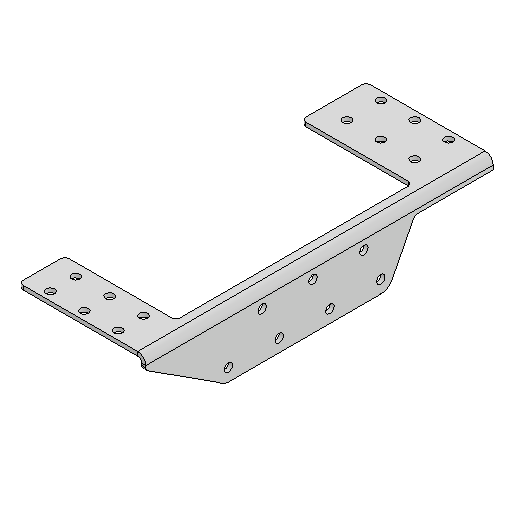
# Autodesk Inventor part: MainDriveMotorToPlateConnector
Saved by Autodesk Inventor 2025 (Build 290162000, 162)
## iProperties
Created: 2024-04-02
Part Number: MainDriveMotorToPlateConnector
Material: Generic
Document SubType Name: Sheet Metal
Designer: seene
Density: 1 g/cm^3
Sheet Metal Rule: Default
Appearance: Default
Mass: 54.1937 g
Surface Area: 394.583 cm^2
Volume: 54.1937 cm^3
Author: seene
Autodesk Inventor part; units mm, degrees
note: some values were not read from the file. Chosen so that the rebuilt part matches the saved one: flange form of "Plate2".
ref_plane "YZ Plane" through (0, 0, 0) normal (1, 0, 0) x (0, 1, 0)
ref_plane "XZ Plane" through (0, 0, 0) normal (0, 1, 0) x (-1, 0, 0)
ref_plane "XY Plane" through (0, 0, 0) normal (0, 0, 1) x (1, 0, 0)
sketch "Sketch1" plane through (0, 0, 0) normal (0, 1, 0) x (-1, 0, 0)
  line L0 (0, 0) -> (95.25, 0)
  line L1 (95.25, 0) -> (95.25, -260.35)
  line L2 (95.25, -260.35) -> (0, -260.35)
  line L3 (0, -260.35) -> (0, 0)
  circle A0 centre (77.8624, -6.35) radius 3.175
  circle A1 centre (77.8624, -25.4) radius 3.175
  circle A2 centre (52.4624, -6.35) radius 3.175
  circle A3 centre (52.4624, -25.4) radius 3.175
  circle A4 centre (27.0624, -6.35) radius 3.175
  circle A5 centre (27.0624, -25.4) radius 3.175
  circle A6 centre (77.8624, -228.6) radius 3.175
  circle A7 centre (77.8624, -254) radius 3.175
  circle A8 centre (52.4624, -228.6) radius 3.175
  circle A9 centre (52.4624, -254) radius 3.175
  circle A10 centre (27.0624, -228.6) radius 3.175
  circle A11 centre (27.0624, -254) radius 3.175
  line L4 (101.24, -208.719) -> (15.24, -208.719) construction
  line L5 (15.24, -208.719) -> (15.24, -37.719) construction
  line L6 (15.24, -37.719) -> (101.24, -37.719) construction
  line L7 (101.24, -37.719) -> (101.24, -208.719) construction
  line L8 (95.25, -211.894) -> (12.065, -211.894)
  line L9 (12.065, -211.894) -> (12.065, -34.544)
  line L10 (12.065, -34.544) -> (95.25, -34.544)
  dimension "d0" = 95.25
  dimension "d2" = 6.35
  dimension "d3" = 6.35
  dimension "d4" = 17.3876
  dimension "d7" = 19.05
  dimension "d10" = 25.4
  dimension "d15" = 25.4
  dimension "d18" = 25.4
  dimension "d21" = 222.25
  dimension "d22" = 6.35
  dimension "d54" = 86
  dimension "d55" = 177.35
  dimension "d56" = 171
  dimension "d57" = 3.175
  dimension "d58" = 34.544
  dimension "d59" = 3.175
  dimension "d60" = 12.065
  measures "d0" distance of L1.end L2.end
  measures "d2" diameter of A0
  measures "d3" distance from line of A0.centre L0
  measures "d4" distance from line of L1 A0.centre
  measures "d7" distance of A0.centre A1.centre
  measures "d10" distance of A0.centre A2.centre
  measures "d15" distance of A6.centre A7.centre
  measures "d18" distance of A6.centre A8.centre
  measures "d21" distance of A6.centre A0.centre
  measures "d22" distance from line of L2 A7.centre
  measures "d54" distance between parallel lines of L5 L7
  measures "d55" distance of L8.end L9.end
  measures "d56" distance of L4.end L5.end
  measures "d57" distance between parallel lines of L4 L8
  measures "d58" distance between parallel lines of L0 L10
  measures "d59" distance between parallel lines of L9 L5
  measures "d60" distance between parallel lines of L3 L9
extrude "Plate1" add sketch "Sketch1" along normal blind 3.048 contours L0 L1 L10 L9 L8 L2 L3
sketch "Sketch2" plane through (-3.048, 3.048, 0) normal (1, 0, 0) x (0, 1, 0)
  line L0 (0, -260.35) -> (0, 0)
  line L1 (0, 0) -> (-50.8, 0)
  line L2 (-50.8, 0) -> (-50.8, -260.35)
  line L3 (-50.8, -260.35) -> (0, -260.35)
  constraints: 6 end point, 1 horizontal, 1 perpendicular, 1 vertical
edge flange "Flange1" height 50.8 angle 90 thickness 3.048 bend radius 3.048 thickness toward (1, 0, 0) relief tear relief width 3.048 relief depth 1.524 edges at (0, 0, -130.175) wall of the first edge with corners at (-3.048, 3.048, -260.35) (-3.048, 3.048, 0) (-3.048, -47.752, 0) (-3.048, -47.752, -260.35)
bend "Bend1"
corner "Corner1"
sketch "Sketch3" plane through (0, -47.752, 0) normal (1, 0, 0) x (0, 0, -1)
  circle A0 centre (87.2198, 37.9611) radius 3.175
  circle A1 centre (61.8198, 12.5611) radius 3.175
  line L0 (0, 0) -> (0, 44.704) projected
  line L1 (260.35, 0) -> (0, 0) projected
  circle A2 centre (99.9198, 12.5611) radius 3.175
  circle A3 centre (138.0198, 12.5611) radius 3.175
  circle A4 centre (176.1198, 12.5611) radius 3.175
  circle A5 centre (125.3198, 37.9611) radius 3.175
  circle A6 centre (163.4198, 37.9611) radius 3.175
  circle A7 centre (61.8198, 12.5611) radius 9.525
  circle A8 centre (176.1198, 12.5611) radius 9.525
  line L2 (61.8198, 3.0361) -> (176.1198, 3.0361)
  line L3 (0, 44.704) -> (260.35, 44.704) projected
  line L4 (260.35, 44.704) -> (260.35, 0) projected
  line L5 (54.3999, 6.5886) -> (0, 41.529)
  line L6 (184.6703, 8.3641) -> (201.5198, 41.529)
  line L7 (201.5198, 41.529) -> (260.35, 41.529)
  point P0 (0, 47.752)
  point P1 (178.7879, 44.704)
  dimension "d34" = 6.35
  dimension "d35" = 25.4
  dimension "d36" = 25.4
  dimension "d37" = 61.8198
  dimension "d40" = 38.1
  dimension "d47" = 38.1
  dimension "d61" = 6.35
  dimension "d62" = 6.35
  dimension "d64" = 3.175
  dimension "d65" = 3.175
  dimension "d66" = 25.4
  constraints: 9 centre point, 8 end point, 4 point on circle, 3 horizontal, 3 point on line, 1 equal radius, 1 parallel, 10 other
  measures "d34" diameter of A0
  measures "d35" horizontal distance of A0.centre A1.centre
  measures "d36" horizontal distance of A0.centre A1.centre
  measures "d37" distance from line of A1.centre L0
  measures "d40" distance of A1.centre A2.centre
  measures "d47" distance of A0.centre A5.centre
  measures "d61" radial gap between concentric circles of A1 A7
  measures "d62" radial gap between concentric circles of A4 A8
  measures "d64" distance between parallel lines of L7 L3
  measures "d65" distance of L5.end L0.end
  measures "d66" horizontal distance of L6.end A4.centre
extrude "Cut1" cut sketch "Sketch3" against normal blind 3.048 contours A0 | A1 | L0 L5 A7 L2 A8 L6 L7 L4 L1 | A2 | A3 | A4 | A5 | A6
fillet "Fillet1" radius 3.175 8 edges at (-95.25, 1.524, 0) (-95.25, 1.524, -34.544) (-12.065, 1.524, -34.544) (-95.25, 1.524, -211.894) (-12.065, 1.524, -211.894) (-95.25, 1.524, -260.35) (-1.524, -6.223, -201.5198) (-1.524, -6.223, 0)
equation "\"d65\" = d64"
equation "\"d52\" = Thickness"
equation "\"d23\" = Thickness"
equation "\"d24\" = BendReliefWidth"
equation "\"d25\" = BendReliefDepth"
equation "\"d26\" = MinimumRemnant"
equation "\"d27\" = TransitionRadius"
equation "\"d30\" = BendRadius"
equation "\"d31\" = CornerReliefSize"
equation "\"d32\" = GapSize"
equation "\"d33\" = JacobiRadiusSize"
equation "\"BendRadius\" = Thickness"
equation "\"BendReliefWidth\" = Thickness"
equation "\"BendReliefDepth\" = 0.5 * Thickness"
equation "\"CornerReliefSize\" = 4 * Thickness"
equation "\"MinimumRemnant\" = 2 * Thickness"
equation "\"TransitionRadius\" = BendRadius"
equation "\"JacobiRadiusSize\" = BendRadius"
equation "\"GapSize\" = Thickness"
equation "\"Thickness\" = 3.048"
body "Solid1"
